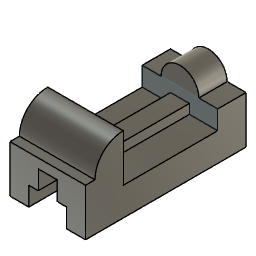
robocon_cad2 v1 (Autodesk Fusion 360 design; units mm, degrees)
Autodesk Fusion 360 part; units mm, degrees
sketch "Sketch1" plane through (0, 0, 0) normal (1, 0, 0) x (0, 1, 0)
  line L0 (8.5, -2.5) -> (-8.5, -2.5)
  line L1 (-8.5, -2.5) -> (-8.5, 2.5)
  line L2 (-8.5, 2.5) -> (8.5, 2.5)
  line L3 (8.5, 2.5) -> (8.5, -2.5)
  line L4 (8.5, -2.5) -> (-8.5, 2.5) construction
  line L5 (-8.5, -2.5) -> (8.5, 2.5) construction
  dimension "d1" = 17
  dimension "d2" = 5
  constraint horizontal L0
  constraint perpendicular L0 L1
  constraint parallel L0 L2
  constraint parallel L1 L3
  constraint coincident L4 origin
  constraint coincident L5 origin
  measures "d1" distance of L1.end L2.end
  measures "d2" distance of L0.end L1.end
extrude "Extrude1" add sketch "Sketch1" against normal blind 8 makes body 1
sketch "Sketch2" plane through (0, 0, 0) normal (1, 0, 0) x (0, 1, 0)
  line L0 (8.5, 2.5) -> (-8.5, 2.5)
  line L1 (-8.5, 2.5) -> (-8.5, -2.5)
  line L2 (-8.5, -2.5) -> (8.5, -2.5)
  line L3 (8.5, -2.5) -> (8.5, 2.5)
  line L4 (-8.5, 2.5) -> (-4.5, 2.5) construction
  line L5 (-4.5, 2.5) -> (5.5, 2.5)
  line L6 (5.5, 2.5) -> (5.5, 0.5)
  line L7 (5.5, 0.5) -> (-4.5, 0.5)
  line L8 (-4.5, 0.5) -> (-4.5, 2.5)
  dimension "d5" = 4
  dimension "d6" = 10
  dimension "d7" = 2
  constraint coincident L0.end L1.start
  constraint perpendicular L1 L4
  constraint horizontal L5
  constraint vertical L6
  constraint horizontal L7
  constraint vertical L8
  measures "d5" distance of L0.end L4.end
  measures "d6" distance of L4.end L5.end
  measures "d7" distance of L4.end L7.end
extrude "Extrude2" cut sketch "Sketch2" against normal up to surface (8 mm away) contours L0 L5 L6 L7 L8 bodies 1
sketch "Sketch3" plane through (0, -8.5, 0) normal (0, -1, 0) x (1, 0, 0)
  line L0 (0, -2.5) -> (0, 2.5)
  line L1 (0, 2.5) -> (-8, 2.5)
  line L2 (-8, 2.5) -> (-8, -2.5)
  line L3 (-8, -2.5) -> (0, -2.5)
  line L4 (0, -2.5) -> (-2, -2.5) construction
  line L5 (-2, -2.5) -> (-2, -0.5)
  line L6 (-2, -0.5) -> (-3, -0.5)
  line L7 (-3, -0.5) -> (-3, 1.5)
  line L8 (-3, 1.5) -> (-5, 1.5)
  line L9 (-5, 1.5) -> (-5, -0.5)
  line L10 (-5, -0.5) -> (-6, -0.5)
  line L11 (-6, -0.5) -> (-6, -2.5)
  dimension "d10" = 2
  dimension "d11" = 2
  dimension "d12" = 2
  dimension "d13" = 2
  constraint coincident L0.start L3.end
  constraint perpendicular L0 L4
  constraint perpendicular L3 L5
  constraint perpendicular L5 L6
  constraint perpendicular L6 L7
  constraint perpendicular L7 L8
  constraint perpendicular L8 L9
  constraint perpendicular L9 L10
  constraint coincident L3 L11.end
  constraint perpendicular L3 L11
  measures "d10" distance of L0.start L4.end
  measures "d11" distance of L4.end L5.end
  measures "d12" distance of L6.end L7.end
  measures "d13" distance of L8.end L9.end
extrude "Extrude3" cut sketch "Sketch3" against normal up to surface (17 mm away) contours L3 L5 L6 L7 L8 L9 L10 L11 bodies 1
sketch "Sketch4" plane through (0, 0, 0.5) normal (0, 0, 1) x (-1, 0, 0)
  line L0 (3, -5.5) -> (3, 4.5)
  line L1 (3, 4.5) -> (0, 4.5)
  line L2 (0, 4.5) -> (0, -5.5)
  line L3 (0, -5.5) -> (3, -5.5)
  line L4 (3, 4.5) -> (5, 4.5)
  line L5 (5, 4.5) -> (5, -5.5)
  line L6 (5, -5.5) -> (3, -5.5)
  line L7 (3, -5.5) -> (3, 4.5)
  dimension "d16" = 2
  dimension "d17" = 10
  constraint horizontal L4
  constraint vertical L5
  constraint horizontal L6
  constraint vertical L7
  constraint coincident L0.end L1.start
  measures "d16" distance of L0.end L4.end
  measures "d17" distance of L0.end L0.start
extrude "Extrude4" add sketch "Sketch4" along normal blind 1 separate body contours L0 L4 L5 L6 L7 makes body 2
sketch "Sketch5" plane through (0, 0, 0) normal (1, 0, 0) x (0, 1, 0)
  line L0 (-4.5, 0.5) -> (-4.5, 2.5)
  line L1 (-4.5, 2.5) -> (-8.5, 2.5)
  line L2 (-8.5, 2.5) -> (-8.5, -2.5)
  line L3 (-8.5, -2.5) -> (8.5, -2.5)
  line L4 (8.5, -2.5) -> (8.5, 2.5)
  line L5 (8.5, 2.5) -> (5.5, 2.5)
  line L6 (5.5, 2.5) -> (5.5, 0.5)
  line L7 (5.5, 0.5) -> (-4.5, 0.5)
  line L8 (-4.5, 2.5) -> (-4.5, 5.5)
  arc A0 (-4.5, 5.5) -> (-7.5, 2.5) centre (-4.5, 2.5) ccw
  dimension "d20" = 3
  constraint coincident L0.end L1.start
  constraint perpendicular L1 L8
  measures "d20" distance of L0.end L8.end
extrude "Extrude5" add sketch "Sketch5" against normal blind 8 contours L1 L8 A0 bodies 1
sketch "Sketch6" plane through (0, 5.5, 0) normal (0, -1, 0) x (1, 0, 0)
  line L0 (-3, 1.5) -> (-3, 0.5)
  line L1 (-3, 0.5) -> (0, 0.5)
  line L2 (0, 0.5) -> (0, 2.5)
  line L3 (0, 2.5) -> (-8, 2.5)
  line L4 (-8, 2.5) -> (-8, 0.5)
  line L5 (-8, 0.5) -> (-5, 0.5)
  line L6 (-5, 0.5) -> (-5, 1.5)
  line L7 (-5, 1.5) -> (-3, 1.5)
sketch "Sketch7" plane through (0, 8.5, 0) normal (0, 1, 0) x (-1, 0, 0)
  line L0 (6, -0.5) -> (6, -2.5)
  line L1 (6, -2.5) -> (8, -2.5)
  line L2 (8, -2.5) -> (8, 2.5)
  line L3 (8, 2.5) -> (0, 2.5)
  line L4 (0, 2.5) -> (0, -2.5)
  line L5 (0, -2.5) -> (2, -2.5)
  line L6 (2, -2.5) -> (2, -0.5)
  line L7 (2, -0.5) -> (3, -0.5)
  line L8 (3, -0.5) -> (3, 1.5)
  line L9 (3, 1.5) -> (5, 1.5)
  line L10 (5, 1.5) -> (5, -0.5)
  line L11 (5, -0.5) -> (6, -0.5)
  arc A0 (6, 2.5) -> (2, 2.5) centre (4, 2.5) ccw
  dimension "d23" = 2
  constraint coincident L3 A0.start
  constraint midpoint L3 A0.centre
  measures "d23" radius of A0
extrude "Extrude6" add sketch "Sketch7" against normal blind 3 contours L3 A0 bodies 1
